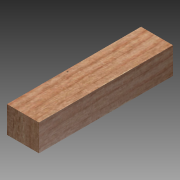
# Autodesk Inventor part: CNC-A- Y-axis support on X-axis
Saved by Autodesk Inventor 2015 (Build 190159000, 159)
## iProperties
Created: 2015-03-25
Part Number: CNC-A- Y-axis support on X-axis
Material: Generic
Document SubType Name: Modeling
Designer: Bangladesh
Density: 1 g/cm^3
Appearance: Default
Author: Bangladesh
Autodesk Inventor part; units mm, degrees
ref_plane "YZ Plane" through (0, 0, 0) normal (1, 0, 0) x (0, 1, 0)
ref_plane "XZ Plane" through (0, 0, 0) normal (0, 1, 0) x (-1, 0, 0)
ref_plane "XY Plane" through (0, 0, 0) normal (0, 0, 1) x (1, 0, 0)
sketch "Sketch1" plane through (0, 0, 0) normal (0, 0, 1) x (1, 0, 0)
  line L0 (-19.05, 15.875) -> (19.05, 15.875)
  line L1 (19.05, 15.875) -> (19.05, -15.875)
  line L2 (19.05, -15.875) -> (-19.05, -15.875)
  line L3 (-19.05, -15.875) -> (-19.05, 15.875)
  line L4 (-19.05, 15.875) -> (19.05, -15.875) construction
  line L5 (19.05, 15.875) -> (-19.05, -15.875) construction
  point P0 (0, 0)
  dimension "d0" = 38.1
  dimension "d1" = 31.75
  constraints: 12 end point, 2 midpoint, 2 parallel, 1 horizontal, 1 perpendicular
  measures "d0" distance of L1.end L2.end
  measures "d1" distance of L0.end L1.end
extrude "Extrusion1" add sketch "Sketch1" along normal mid plane 160
body "Solid1"
